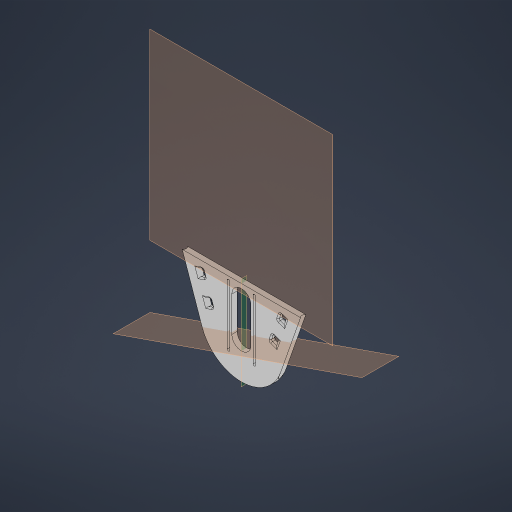
# Autodesk Inventor part: StepperBoard
Saved by Autodesk Inventor 2024 (Build 280153000, 153)
## iProperties
Created: 2023-10-21
Part Number: StepperBoard
Material: Generic
Document SubType Name: Modeling
Designer: range
Density: 1 g/cm^3
Appearance: Default
Author: range
Autodesk Inventor part; units mm, degrees
ref_plane "YZ Plane" through (0, 0, 0) normal (1, 0, 0) x (0, 1, 0)
ref_plane "XZ Plane" through (0, 0, 0) normal (0, 1, 0) x (-1, 0, 0)
ref_plane "XY Plane" through (0, 0, 0) normal (0, 0, 1) x (1, 0, 0)
ref_plane "Work Plane1" through (0, 0, 0) normal (0, 0, 1) x (1, 0, 0)
sketch "Sketch1" plane through (0, 0, 0) normal (0, 0, 1) x (1, 0, 0)
  line L0 (-47.2324, -168.8042) -> (-94.4649, -32.8084) projected
  line L1 (71.1287, -100) -> (32.49, -100) projected
  line L2 (32.49, -100) -> (71.1287, -100) projected
  circle A0 centre (0, -152.4) radius 50 projected
  line L3 (13.994, -176.784) -> (13.994, -159.004) projected
  arc A1 (13.994, -176.784) -> (16.994, -176.784) centre (15.494, -176.784) ccw projected
  line L4 (16.994, -159.004) -> (16.994, -176.784) projected
  arc A2 (16.994, -159.004) -> (13.994, -159.004) centre (15.494, -159.004) ccw projected
  line L5 (13.994, -145.796) -> (13.994, -128.016) projected
  arc A3 (13.994, -145.796) -> (16.994, -145.796) centre (15.494, -145.796) ccw projected
  line L6 (16.994, -128.016) -> (16.994, -145.796) projected
  arc A4 (16.994, -128.016) -> (13.994, -128.016) centre (15.494, -128.016) ccw projected
  line L7 (13.994, -145.796) -> (13.994, -128.016) projected
  arc A5 (-16.994, -176.784) -> (-13.994, -176.784) centre (-15.494, -176.784) ccw projected
  line L8 (-16.994, -176.784) -> (-16.994, -159.004) projected
  line L9 (-13.994, -159.004) -> (-13.994, -176.784) projected
  arc A6 (-13.994, -159.004) -> (-16.994, -159.004) centre (-15.494, -159.004) ccw projected
  arc A7 (-16.994, -145.796) -> (-13.994, -145.796) centre (-15.494, -145.796) ccw projected
  line L10 (-16.994, -145.796) -> (-16.994, -128.016) projected
  line L11 (-13.994, -128.016) -> (-13.994, -145.796) projected
  arc A8 (-13.994, -128.016) -> (-16.994, -128.016) centre (-15.494, -128.016) ccw projected
  arc A9 (11.493, -146.05) -> (-11.493, -146.05) centre (0, -146.05) ccw projected
  arc A10 (-11.493, -158.75) -> (11.493, -158.75) centre (0, -158.75) ccw projected
  circle A11 centre (0, -152.4) radius 50 projected
  line L12 (-47.2324, -168.8042) -> (-94.4649, -32.8084) projected
  line L13 (47.2324, -168.8042) -> (94.4649, -32.8084) projected
  line L14 (-94.4649, -32.8084) -> (94.4649, -32.8084)
  line L15 (-11.493, -158.75) -> (-11.493, -146.05)
  line L16 (11.493, -158.75) -> (11.493, -146.05)
  line L17 (-34.4196, -142.831) -> (-40.4181, -144.9143) projected
  line L18 (-37.3363, -134.4331) -> (-43.3348, -136.5164) projected
  line L19 (-43.5863, -116.4375) -> (-49.5848, -118.5208) projected
  line L20 (-46.5029, -108.0396) -> (-52.5015, -110.1229) projected
  line L21 (43.5863, -116.4375) -> (49.5848, -118.5208) projected
  line L22 (46.5029, -108.0396) -> (52.5015, -110.1229) projected
  line L23 (37.3363, -134.4331) -> (43.3348, -136.5164) projected
  line L24 (34.4196, -142.831) -> (40.4181, -144.9143) projected
  circle A12 centre (0, -152.4) radius 35.725 projected
  line L25 (-56.9859, -19.7917) -> (-9.7535, -155.7875) projected
  line L26 (56.9859, -19.7917) -> (9.7535, -155.7875) projected
  line L27 (40.4181, -144.9143) -> (52.5015, -110.1229)
  line L28 (46.5029, -108.0396) -> (34.4196, -142.831)
  line L29 (-52.5015, -110.1229) -> (-40.4181, -144.9143)
  line L30 (-34.4196, -142.831) -> (-46.5029, -108.0396)
  line L31 (-32.49, -100) -> (-71.1287, -100) projected
  line L32 (-32.49, -100) -> (32.49, -100)
  line L33 (-15.494, -128.016) -> (-15.494, -104.8612) construction
  line L34 (-16.994, -128.016) -> (-16.994, -104.8612)
  line L35 (-13.994, -104.8612) -> (-13.994, -128.016)
  arc A13 (-16.994, -128.016) -> (-13.994, -128.016) centre (-15.494, -128.016) ccw
  arc A14 (-13.994, -104.8612) -> (-16.994, -104.8612) centre (-15.494, -104.8612) ccw
  line L36 (15.494, -128.016) -> (15.494, -104.8612) construction
  line L37 (13.994, -128.016) -> (13.994, -104.8612)
  line L38 (16.994, -104.8612) -> (16.994, -128.016)
  arc A15 (13.994, -128.016) -> (16.994, -128.016) centre (15.494, -128.016) ccw
  arc A16 (16.994, -104.8612) -> (13.994, -104.8612) centre (15.494, -104.8612) ccw
  line L39 (-15.494, -159.004) -> (-15.494, -145.796) construction
  line L40 (-16.994, -159.004) -> (-16.994, -145.796)
  line L41 (-13.994, -145.796) -> (-13.994, -159.004)
  arc A17 (-16.994, -159.004) -> (-13.994, -159.004) centre (-15.494, -159.004) ccw
  arc A18 (-13.994, -145.796) -> (-16.994, -145.796) centre (-15.494, -145.796) ccw
  line L42 (15.494, -159.004) -> (15.494, -145.796) construction
  line L43 (13.994, -159.004) -> (13.994, -145.796)
  line L44 (16.994, -145.796) -> (16.994, -159.004)
  arc A19 (13.994, -159.004) -> (16.994, -159.004) centre (15.494, -159.004) ccw
  arc A20 (16.994, -145.796) -> (13.994, -145.796) centre (15.494, -145.796) ccw
  line L45 (0, -146.05) -> (0, -116.675) construction
  line L46 (-11.493, -146.05) -> (-11.493, -116.675)
  line L47 (11.493, -116.675) -> (11.493, -146.05)
  arc A21 (-11.493, -146.05) -> (11.493, -146.05) centre (0, -146.05) ccw
  arc A22 (11.493, -116.675) -> (-11.493, -116.675) centre (0, -116.675) ccw
  point P0 (0, 0)
  point P1 (-9.7535, -155.7875)
  point P2 (20.9741, -123.4801)
  point P3 (-20.9741, -123.4801)
  point P4 (29.1289, -100)
  point P5 (25.8041, -109.5731)
  point P6 (-25.8041, -109.5731)
  point P7 (-29.1289, -100)
  point P8 (29.1289, -100)
  point P9 (29.1289, -100)
  point P10 (-29.1289, -100)
  point P11 (52.4651, -32.8084)
  point P12 (-52.4651, -32.8084)
  point P13 (-15.494, -116.4386)
  point P14 (15.494, -116.4386)
  point P15 (-15.494, -152.4)
  point P16 (15.494, -152.4)
  point P17 (0, -131.3625)
  constraints: 56 end point, 23 point on circle, 20 tangent, 10 centre point, 8 parallel, 5 midpoint, 4 vertical, 2 horizontal, 1 perpendicular, 3 other
extrude "Extrusion1" add sketch "Sketch1" against normal blind 6.35 contours A0 L29 L17 A12 L24 L27 | L0 L31 L32 L25 A0 L30 L20 L29 | A0 L27 L22 L28 L26 L32 L1 L13 | L29 L19 L30 A0 | A0 L30 L18 L29 | A0 L25 A12 L30 | L32 L26 A0 L38 A16 A14 L34 L25 | L27 L23 L28 A0 | A0 L28 L21 L27 | A0 L34 A12 L25 | L28 A12 L26 A0 | L25 L10 L40 L8 A5 L9 L41 L11 L15 A10 L16 L26 L5 L43 L3 A1 L4 L44 L6 A12 | A12 L34 L10 L25 | L26 A12 L38 A0 | A0 A16 L37 A12 L47 A22 L46 L35 A14 | L26 L6 L38 A12 | A12 L46 L15 L25 L11 L35 | L37 L5 L26 L16 L47 A12
fillet "Fillet1" [suppressed]
ref_plane "Work Plane2" through (-47.2324, -168.8042, -6.35) normal (-0.328084, 0.9446486, 0) x (0, 0, 1)
sketch "Sketch2" plane through (-47.2324, -168.8042, -6.35) normal (-0.328084, 0.9446486, 0) x (0, 0, 1)
  arc A0 (6.35, 0) -> (0, 0) centre (3.175, -2.3917) ccw projected
  line L0 (0, 97.2324) -> (0, 97.2324) projected
  line L1 (6.35, 0) -> (0, 0)
  point P0 (6.35, 100)
  point P1 (0, 89.2361)
  constraints: 2 end point, 1 horizontal, 1 other
extrude "Extrusion2" cut sketch "Sketch2" along normal through all both and the other way through all
fillet "Fillet2" radius 3.175 8 edges at (-51.0431, -114.3219, 0) (-51.0431, -114.3219, -6.35) (-41.8765, -140.7154, 0) (-41.8765, -140.7154, -6.35) (51.0431, -114.3219, 0) (51.0431, -114.3219, -6.35) (41.8765, -140.7154, 0) (41.8765, -140.7154, -6.35)
fillet "Fillet2" radius 1.5875 32 edges at (49.5022, -109.0813, 0) (45.0446, -112.2386, 0) (46.5855, -117.4792, 0) (49.5022, -109.0813, -6.35) (46.5855, -117.4792, -6.35) (45.0446, -112.2386, -6.35) (43.5863, -116.4375, -3.175) (46.5029, -108.0396, -3.175) (40.3355, -135.4747, 0) (35.8779, -138.632, 0) (37.4189, -143.8727, 0) (34.4196, -142.831, -3.175) (37.3363, -134.4331, -3.175) (40.3355, -135.4747, -6.35) (35.8779, -138.632, -6.35) (37.4189, -143.8727, -6.35) (-46.5029, -108.0396, -3.175) (-49.5022, -109.0813, -6.35) (-45.0446, -112.2386, -6.35) (-46.5855, -117.4792, -6.35) (-46.5855, -117.4792, 0) (-49.5022, -109.0813, 0) (-45.0446, -112.2386, 0) (-43.5863, -116.4375, -3.175) (-40.3355, -135.4747, -6.35) (-35.8779, -138.632, -6.35) (-37.4189, -143.8727, -6.35) (-34.4196, -142.831, -3.175) (-37.3363, -134.4331, -3.175) (-40.3355, -135.4747, 0) (-35.8779, -138.632, 0) (-37.4189, -143.8727, 0)
ref_plane "Work Plane3" through (0, -158.75, 0) normal (-1, 0, 0) x (0, 0, 1)
mirror "Mirror1" about plane through (0, -158.75, 0) normal (-1, 0, 0) of "Extrusion2"
body "Solid1"
